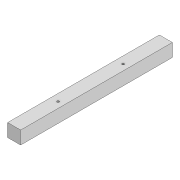
# Autodesk Inventor part: Träger vorne
Saved by Autodesk Inventor 2020 (Build 240168000, 168)
## iProperties
Created: 2021-06-23
Part Number: Träger vorne
Material: Generisch
Document SubType Name: Modeling
Designer: mike8
Density: 1 g/cm^3
Appearance: Vorgabe
Author: mike8
Autodesk Inventor part; units mm, degrees
ref_plane "YZ Plane" through (0, 0, 0) normal (1, 0, 0) x (0, 1, 0)
ref_plane "XZ Plane" through (0, 0, 0) normal (0, 1, 0) x (-1, 0, 0)
ref_plane "XY Plane" through (0, 0, 0) normal (0, 0, 1) x (1, 0, 0)
sketch "Skizze1" plane through (0, 0, 0) normal (0, 0, 1) x (1, 0, 0)
  line L0 (-27.9018, 0) -> (14.0982, 0) projected
  line L1 (0, -20.5399) -> (0, 21.4601) projected
  line L2 (-21.9018, 15.4601) -> (8.0982, 15.4601)
  line L3 (8.0982, 15.4601) -> (8.0982, -14.5399)
  line L4 (8.0982, -14.5399) -> (-21.9018, -14.5399)
  line L5 (-21.9018, -14.5399) -> (-21.9018, 15.4601)
  point P0 (0, 0)
  dimension "d0" = 30
  dimension "d1" = 30
  constraints: 8 end point, 2 parallel, 1 horizontal, 1 perpendicular
  measures "d0" distance of L4.end L2.start
  measures "d1" distance of L2.start L2.end
extrude "Extrusion1" add sketch "Skizze1" along normal blind 350
sketch "Skizze2" plane through (-21.9018, 15.4601, 0) normal (0, 1, 0) x (1, 0, 0)
  line L0 (30, 0) -> (0, 0) projected
  line L1 (30, -350) -> (0, -350) projected
  point P0 (21.9018, 0)
  point P1 (16.3934, -100)
  point P2 (16.3934, -250)
  dimension "d4" = 100
  dimension "d5" = 100
  measures "d4" distance from line of L0 point (16.393, -100)
  measures "d5" distance from line of L1 point (16.393, -250)
hole "Bohrung1" at (-5.5084, 15.4601, 100) at (-5.5084, 15.4601, 250) direction (0, -1, 0) diameter 5 end through all
